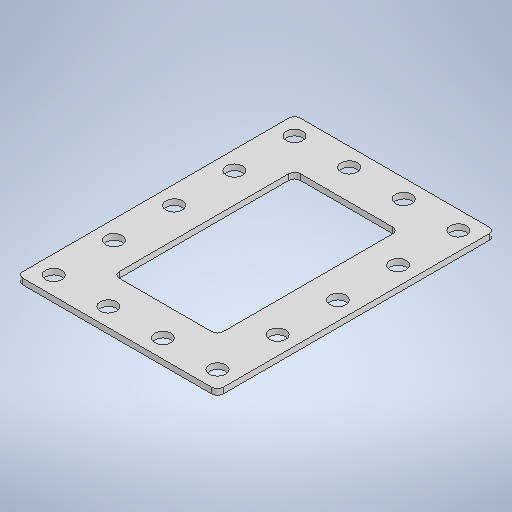
# Autodesk Inventor part: PRS 9606 charging flange round_D1200
Saved by Autodesk Inventor 2026.2 (Build 302298000, 298)
## iProperties
Created: 2025-02-13
Part Number: PRS 9606 charging flange round_D1200
Material: Steel
Document SubType Name: Sheet Metal
Designer: admin
Mass: 2466.79 g
Surface Area: 934.137 cm^2
Volume: 314.241 cm^3
Density: 7.85 g/cm^3
Flat Pattern Width: 28.8 cm
Flat Pattern Length: 20.8 cm
Flat Pattern Area: 599.04 cm^2
Sheet Metal Rule: AISI304 4mm Die 32
Sheet Metal Width: 288,000 mm
Sheet Metal Length: 208,000 mm
Sheet Metal Area: 59904,000 mm^2
Appearance: Default
Author: pokla
Autodesk Inventor part; units mm, degrees
ref_plane "YZ Plane" through (0, 0, 0) normal (1, 0, 0) x (0, 1, 0)
ref_plane "XZ Plane" through (0, 0, 0) normal (0, 1, 0) x (-1, 0, 0)
ref_plane "XY Plane" through (0, 0, 0) normal (0, 0, 1) x (1, 0, 0)
sketch "Sketch2" plane through (0, 0, 0) normal (0, 0, 1) x (1, 0, 0)
  line L0 (-54, -94) -> (54, -94)
  line L1 (54, -94) -> (54, 94)
  line L2 (54, 94) -> (-54, 94)
  line L3 (-54, 94) -> (-54, -94)
  line L4 (-54, -94) -> (54, 94) construction
  line L5 (54, -94) -> (-54, 94) construction
  line L6 (-104, -144) -> (104, -144)
  line L7 (104, -144) -> (104, 144)
  line L8 (104, 144) -> (-104, 144)
  line L9 (-104, 144) -> (-104, -144)
  point P0 (0, 0)
  dimension "d29" = 108
  dimension "d30" = 188
  dimension "d31" = 50
  measures "d29" distance of L2.end L1.end
  measures "d30" distance of L1.end L0.end
  measures "d31" distance between parallel lines of L3 L9
extrude "Plate2" add sketch "Sketch2" along normal blind 6
sketch "Sketch5" plane through (0, 0, 6) normal (0, 0, 1) x (1, 0, 0)
  line L0 (54, 94) -> (54, -94) construction
  line L1 (54, -94) -> (-54, -94) construction
  line L2 (-54, -94) -> (-54, 94) construction
  line L3 (-54, 94) -> (54, 94) construction
  line L4 (104, -144) -> (-104, -144) construction
  line L5 (104, 144) -> (104, -144) construction
  line L6 (-104, 144) -> (104, 144) construction
  line L7 (-104, -144) -> (-104, 144) construction
  line L8 (-85, 125) -> (85, 125) construction
  line L9 (85, 125) -> (85, -125) construction
  line L10 (85, -125) -> (-85, -125) construction
  line L11 (-85, -125) -> (-85, 125) construction
  line L12 (-54, 0) -> (54, 0) construction
  line L13 (0, 94) -> (0, -94)
  point P0 (0, 0)
  point P1 (0, -125)
  point P2 (-85, 62.5)
  point P3 (-85, 0)
  point P4 (-85, -62.5)
  point P5 (-28.3333, -125)
  point P6 (28.3333, -125)
  point P7 (85, -62.5)
  point P8 (85, 0)
  point P9 (85, 62.5)
  point P10 (28.3333, 125)
  point P11 (-28.3333, 125)
  dimension "d34" = 19
  dimension "d49" = 62.5
  dimension "d50" = 62.5
  dimension "d51" = 56.6667
  dimension "d52" = 56.6667
  dimension "d53" = 56.6667
  constraints: 12 end point, 8 point on line, 7 midpoint, 4 coincident, 3 symmetric about line, 2 vertical alignment, 1 horizontal alignment, 3 other
  measures "d34" distance between parallel lines of L4 L10
  measures "d49" distance of point (-85, 62.5) point (-85, 125)
  measures "d50" distance of point (-85, 0) point (-85, 62.5)
  measures "d51" distance of point (-28.333, 125) point (-85, 125)
  measures "d52" distance of point (28.333, 125) point (-28.333, 125)
  measures "d53" distance of point (85, 125) point (28.333, 125)
fillet "Corner Round1" radius 6 8 edges at (-104, -144, 3) (-104, 144, 3) (104, 144, 3) (104, -144, 3) (54, -94, 3) (-54, -94, 3) (-54, 94, 3) (54, 94, 3)
hole "Hole1" at (-85, 125, 6) at (-85, 62.5, 6) at (-85, 0, 6) at (-85, -62.5, 6) at (-85, -125, 6) at (-28.3333, -125, 6) at (28.3333, -125, 6) at (85, -125, 6) at (85, -62.5, 6) at (85, 0, 6) at (85, 62.5, 6) at (85, 125, 6) at (28.3333, 125, 6) at (-28.3333, 125, 6) direction (0, 0, -1) diameter 17 end through all
equation "\"d49\" = d50"
equation "\"d51\" = d53"
equation "\"d52\" = d53"
equation "\"d29\" = ChargingHatch_hight - 2 * Thickness"
equation "\"d30\" = ChargingHatch_width - 2 * Thickness"
equation "\"d59\" = Thickness"
equation "\"d14\" = Thickness"
equation "\"BendReliefWidth\" = Thickness"
equation "\"BendReliefDepth\" = 0.5 * Thickness"
equation "\"CornerReliefSize\" = 4 * Thickness"
equation "\"MinimumRemnant\" = 2 * Thickness"
equation "\"TransitionRadius\" = BendRadius"
equation "\"JacobiRadiusSize\" = BendRadius"
equation "\"GapSize\" = Thickness"
equation "\"ChargingHatch_hight\" = 120"
equation "\"Thickness\" = 6"
equation "\"ChargingHatch_width\" = 200"
equation "\"BendRadius\" = 6"
body "Solid3"
